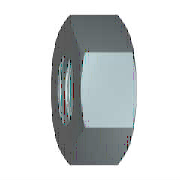
# Autodesk Inventor part: CNS 3129 - M 2
Saved by Autodesk Inventor 2017 (Build 210142000, 142)
## iProperties
IsCustomPart: 0
Created: 2016-02-22
Part Number: CNS 3129 - M 2
Material: Steel, Mild
Description: Hex Nut
Document SubType Name: Modeling
Standard: CNS 3129
Designer: Admin
Standards Organization: CNS
Language: en-US
Size Designation: M 2
Categories: <MemberInstance><Categories><Category DisplayName="Fasteners" InternalName="e4da775c-781d-43d5-af7c-5136215cf5a6" Mnemonic="FSTN"><Category DisplayName="Nuts" InternalName="e37c7a56-0470-4688-8db4-b4d75d611516" Mnemonic="NUT"><CategoryParameter DisplayName="Thread Designation" InternalName="10aefdba-3783-44b8-becc-0feae870ab73" Mnemonic="thrdesign"/><CategoryParameter DisplayName="Thread Series Designation" InternalName="17a0ae10-6923-48a9-85c7-ae9b76790e6f" Mnemonic="thrserdsgn"/><CategoryParameter DisplayName="Thread Type" InternalName="205c6614-02f1-43b1-b704-b331415a8186" Mnemonic="thrtype"/><CategoryParameter DisplayName="Nominal Diameter Designation" InternalName="39406bc0-754a-4a9f-8c64-e1bba9d40b8a" Mnemonic="nomdiadesig"/><CategoryParameter DisplayName="Height" InternalName="5579c84d-d692-41f2-8996-171d03c19b53" Mnemonic="nheig"/><CategoryParameter DisplayName="Thread Class" InternalName="9b95427d-7bb5-461a-8a3e-4650073a592b" Mnemonic="thrclss"/><CategoryParameter DisplayName="Thread Pitch" InternalName="bd2c58b1-df6d-45e3-8bf7-4a0997b15b95" Mnemonic="pitch1"/><CategoryParameter DisplayName="Nominal Diameter" InternalName="d6e3b243-37ab-4432-98ea-592d296d3a46" Mnemonic="nomdia"/><CategoryParameter DisplayName="Threads per Unit" InternalName="e2e4d09d-bc7f-4af6-8086-8693b8d97bcd" Mnemonic="thrperunit1"/><Category DisplayName="Hex" InternalName="73d9c703-2233-4460-907f-38a87f245fbb" Mnemonic="PLNUT"><CategoryParameter DisplayName="Width Across Corners" InternalName="3db1d29f-9506-4e4b-a66f-416ec1d0915f" Mnemonic="wacor"/><CategoryParameter DisplayName="Type" InternalName="4e484966-9917-44a5-bcb5-b45bf8fff7e8" Mnemonic="type"/><CategoryParameter DisplayName="Property Class" InternalName="bcb84129-2a2e-4fb9-8398-d46bb849f471" Mnemonic="propclss"/></Category></Category></Category><Category DisplayName="DataType" InternalName="23b78d0f-2648-40c6-8793-ca6db495c9e8" Mnemonic="DATATYPE"><CategoryParameter DisplayName="DisplayName" InternalName="05415f3d-3907-474b-a020-eb9d644f4cf3" Mnemonic="DISPLAYNAME"/><CategoryParameter DisplayName="Standard" InternalName="0c0a119c-1e12-4c84-803f-101930972f5e" Mnemonic="STANDARD"/><CategoryParameter DisplayName="Description" InternalName="13903e3d-64b1-4950-80da-f627842ea37f" Mnemonic="DESCRIPTION"/><CategoryParameter DisplayName="Designation" InternalName="2675968c-4ce5-49e0-a4f5-552d29089031" Mnemonic="DESIGNATION"/><CategoryParameter DisplayName="Default Row" InternalName="2af9ec52-faaa-4026-b378-f9fa4afca842" Mnemonic="DEFAULTROW"/><CategoryParameter DisplayName="Folder Name" InternalName="3f06958e-8713-4116-9be7-ed6184ecc97b" Mnemonic="FOLDERNAME"/><CategoryParameter DisplayName="Revision Guid" InternalName="45a75005-10b1-4dfc-8d6d-dfe629f0b93c" Mnemonic="REVISIONGUID"/><CategoryParameter DisplayName="FileName" InternalName="8b46a4cc-9585-4fed-90c3-899f57e09a73" Mnemonic="FILENAME"/><CategoryParameter DisplayName="StdsOrg" InternalName="8f5914e1-4693-403f-8ab5-d37768198c9d" Mnemonic="STDSORG"/><CategoryParameter DisplayName="Family Version" InternalName="914462f6-6e19-4b14-ba84-155b9680b1d0" Mnemonic="FAMILYREVISION"/><CategoryParameter DisplayName="Standard Revision" InternalName="91d5a463-65c2-4fde-b823-3b7fea5e8e17" Mnemonic="STANDARDREVISION"/><CategoryParameter DisplayName="Member Revision" InternalName="a65d44b9-392f-4f4f-857b-e4b3d54996fe" Mnemonic="MEMBERREVISION"/><CategoryParameter DisplayName="ClipFormat" InternalName="bc51e27b-3422-4e78-93ef-cec197ddf230" Mnemonic="CLIPFORMAT"/><CategoryParameter DisplayName="Manufacturer" InternalName="cd6c7a72-a28a-4e50-99a9-2c7f4e13e5ad" Mnemonic="MANUFACTURER"/><CategoryParameter DisplayName="InternalName" InternalName="cf1d0246-76d9-4b4a-8305-fa0409afb5c1" Mnemonic="INTERNALNAME"/><CategoryParameter DisplayName="IsMetric" InternalName="e2385c5b-1ea4-4823-96a8-8de651266ec3" Mnemonic="ISMETRIC"/><Category DisplayName="Part" InternalName="c0e0b642-3bcb-4cc8-9e80-f96d35c4afa4" Mnemonic="PART"><CategoryParameter DisplayName="Part Number" InternalName="016b6077-bfbe-49bd-92c9-d8d59c39c941" Mnemonic="PARTNUMBER"/><CategoryParameter DisplayName="Stock Number" InternalName="4dba7c1c-e26c-444e-836c-b08b433409a8" Mnemonic="STOCKNUMBER"/><CategoryParameter DisplayName="Material Key" InternalName="5c9a8adb-dd2b-4535-b97f-0a94a95fe41f" Mnemonic="MATERIALKEY"/><CategoryParameter DisplayName="Material" InternalName="818a152a-d3c3-49ca-80ee-df7d91421b8e" Mnemonic="MATERIAL"/></Category></Category><Category DisplayName="LegacyMap" InternalName="cd87c42b-3e48-431e-b5c0-1cbeb14dfe77" Mnemonic="LEGACYMAP"><CategoryParameter DisplayName="unique DA member ID" InternalName="0918ad47-427f-4fed-ae26-24c81c58f590" Mnemonic="DACOOKIE"/><CategoryParameter DisplayName="Merge11 ID" InternalName="0ee8fb18-e2ed-4f39-96f6-1f4b5f50aa71" Mnemonic="MERGE11"/><CategoryParameter DisplayName="unique CC member ID" InternalName="5193edd4-b2b0-4ab4-9d54-de900eee34e0" Mnemonic="CCCOOKIE"/><CategoryParameter DisplayName="Split ID" InternalName="72b5c83c-be7f-45c4-ae51-9160ea6deb26" Mnemonic="SPLIT"/><CategoryParameter DisplayName="MemberID" InternalName="8e5e0294-fc51-4c8f-b3d7-003dc5ed94f6" Mnemonic="MEMBERID"/><CategoryParameter DisplayName="CatalogName" InternalName="d99d1e27-aa94-4de2-af4c-c348882a6f4f" Mnemonic="CATALOGNAME"/><CategoryParameter DisplayName="FamilyNumber" InternalName="e705e1f4-09cb-413e-91f9-551b4188271e" Mnemonic="FAMILYNUMBER"/></Category></Categories><FamilyTemplate Id="no0010"><FamilyTemplateParameters><FamilyTemplateParameter ObjectType="kUserParameterObject" ValueType="xs:double" Id="1" ObjectReferenceKey="GUL"/><FamilyTemplateParameter ObjectType="kUserParameterObject" ValueType="xs:double" Id="2" ObjectReferenceKey="KOH"/><FamilyTemplateParameter ObjectType="kUserParameterObject" ValueType="xs:double" Id="3" ObjectReferenceKey="TPU"/><FamilyTemplateParameter ObjectType="kUserParameterObject" ValueType="xs:double" Id="4" ObjectReferenceKey="GD1"/><FamilyTemplateParameter ObjectType="kUserParameterObject" ValueType="xs:double" Id="5" ObjectReferenceKey="SW01"/><FamilyTemplateParameter ObjectType="kUserParameterObject" ValueType="xs:double" Id="6" ObjectReferenceKey="THREADDIA"/><FamilyTemplateParameter ObjectType="kUserParameterObject" ValueType="xs:double" Id="7" ObjectReferenceKey="SW"/><FamilyTemplateParameter ObjectType="kUserParameterObject" ValueType="xs:double" Id="8" ObjectReferenceKey="ANG2"/><FamilyTemplateParameter ObjectType="kUserParameterObject" ValueType="xs:double" Id="9" ObjectReferenceKey="ANG1"/><FamilyTemplateParameter ObjectType="kUserParameterObject" ValueType="xs:double" Id="10" ObjectReferenceKey="TOA"/><FamilyTemplateParameter ObjectType="kUserParameterObject" ValueType="xs:double" Id="11" ObjectReferenceKey="PTC"/><FamilyTemplateParameter ObjectType="kUserParameterObject" ValueType="xs:double" Id="12" ObjectReferenceKey="NND"/><FamilyTemplateParameter ObjectType="kUserParameterObject" ValueType="xs:double" Id="13" ObjectReferenceKey="E0"/><FamilyTemplateParameter ObjectType="kUserParameterObject" ValueType="xs:double" Id="14" ObjectReferenceKey="SW0"/><FamilyTemplateParameter ObjectType="kUserParameterObject" ValueType="xs:double" Id="15" ObjectReferenceKey="GAL"/><FamilyTemplateParameter ObjectType="kPropertyObject" ValueType="xs:string" Id="100" ObjectReferenceKey="{32853F0F-3444-11d1-9E93-0060B03C1CA6}" SubObjectId="52"/><FamilyTemplateParameter ObjectType="kPropertyObject" ValueType="xs:string" Id="105" ObjectReferenceKey="{32853F0F-3444-11d1-9E93-0060B03C1CA6}" SubObjectId="5"/><FamilyTemplateParameter ObjectType="kPartComponentDefinitionObject" ValueType="xs:string" Id="110" SubObjectId="Material"/><FamilyTemplateParameter ObjectType="kThreadFeatureObject" ValueType="xs:structure" Id="300" ObjectReferenceKey="1002000010000000ba090000000000008000000000000000" SubObjectId="ThreadInfo"><FamilyTemplateParameter ObjectType="" ValueType="xs:string" Id="301" SubObjectId="ThreadDesignation"/><FamilyTemplateParameter ObjectType="" ValueType="xs:string" Id="302" SubObjectId="ThreadClass"/><FamilyTemplateParameter ObjectType="" ValueType="xs:string" Id="303" SubObjectId="ThreadType"/></FamilyTemplateParameter></FamilyTemplateParameters></FamilyTemplate><CategoryParameterMap><ParamToTemplateMap><ParamToTemplate CategoryParameter="//CategoryParameter[@InternalName='05415f3d-3907-474b-a020-eb9d644f4cf3']" ConstantValue="CNS 3129"/><ParamToTemplate CategoryParameter="//CategoryParameter[@InternalName='cf1d0246-76d9-4b4a-8305-fa0409afb5c1']" ConstantValue="5d0b1584-d28e-4f5c-b995-5fb680a39008"/><ParamToTemplate CategoryParameter="//CategoryParameter[@InternalName='3f06958e-8713-4116-9be7-ed6184ecc97b']" ConstantValue="CNS 3129"/><ParamToTemplate CategoryParameter="//CategoryParameter[@InternalName='914462f6-6e19-4b14-ba84-155b9680b1d0']" ConstantValue="10"/><ParamToTemplate CategoryParameter="//CategoryParameter[@InternalName='bc51e27b-3422-4e78-93ef-cec197ddf230']" ConstantValue="CF_INVENTOR.STDPARTS"/><ParamToTemplate CategoryParameter="//CategoryParameter[@InternalName='e2385c5b-1ea4-4823-96a8-8de651266ec3']" ConstantValue="true"/><ParamToTemplate CategoryParameter="//CategoryParameter[@InternalName='13903e3d-64b1-4950-80da-f627842ea37f']" ConstantValue="Hex Nut"/><ParamToTemplate CategoryParameter="//CategoryParameter[@InternalName='8f5914e1-4693-403f-8ab5-d37768198c9d']" ConstantValue="CNS"/><ParamToTemplate CategoryParameter="//CategoryParameter[@InternalName='0c0a119c-1e12-4c84-803f-101930972f5e']" ConstantValue="CNS 3129"/><ParamToTemplate CategoryParameter="//CategoryParameter[@InternalName='cd6c7a72-a28a-4e50-99a9-2c7f4e13e5ad']" TemplateParameter="104"/><ParamToTemplate CategoryParameter="//CategoryParameter[@InternalName='91d5a463-65c2-4fde-b823-3b7fea5e8e17']" TemplateParameter="103"/><ParamToTemplate CategoryParameter="//CategoryParameter[@InternalName='45a75005-10b1-4dfc-8d6d-dfe629f0b93c']" ConstantValue="ca1287fc-ef04-4131-a459-e0ad3082d8c4"/><ParamToTemplate CategoryParameter="//CategoryParameter[@InternalName='2af9ec52-faaa-4026-b378-f9fa4afca842']" ConstantValue="10"/><ParamToTemplate CategoryParameter="//CategoryParameter[@InternalName='d99d1e27-aa94-4de2-af4c-c348882a6f4f']" ConstantValue="CNS"/><ParamToTemplate CategoryParameter="//CategoryParameter[@InternalName='8b46a4cc-9585-4fed-90c3-899f57e09a73']" ConstantValue="CNS 3129 - M 2 x 0.4"/><ParamToTemplate CategoryParameter="//CategoryParameter[@InternalName='a65d44b9-392f-4f4f-857b-e4b3d54996fe']" ConstantValue="a0c9818c-55a9-4959-93a9-f48d9538dd43"/><ParamToTemplate CategoryParameter="//CategoryParameter[@InternalName='9b95427d-7bb5-461a-8a3e-4650073a592b']" ConstantValue="6H"/><ParamToTemplate CategoryParameter="//CategoryParameter[@InternalName='17a0ae10-6923-48a9-85c7-ae9b76790e6f']" ConstantValue="Regular Thread"/><ParamToTemplate CategoryParameter="//CategoryParameter[@InternalName='39406bc0-754a-4a9f-8c64-e1bba9d40b8a']" ConstantValue="M2"/><ParamToTemplate CategoryParameter="//CategoryParameter[@InternalName='205c6614-02f1-43b1-b704-b331415a8186']" ConstantValue="ISO Metric Profile"/><ParamToTemplate CategoryParameter="//CategoryParameter[@InternalName='e705e1f4-09cb-413e-91f9-551b4188271e']" ConstantValue="53"/><ParamToTemplate CategoryParameter="//CategoryParameter[@InternalName='8e5e0294-fc51-4c8f-b3d7-003dc5ed94f6']" ConstantValue="30"/><ParamToTemplate CategoryParameter="//CategoryParameter[@InternalName='2675968c-4ce5-49e0-a4f5-552d29089031']" TemplateParameter="100"/><ParamToTemplate CategoryParameter="//CategoryParameter[@InternalName='3db1d29f-9506-4e4b-a66f-416ec1d0915f']" TemplateParameter="13"/><ParamToTemplate CategoryParameter="//CategoryParameter[@InternalName='5579c84d-d692-41f2-8996-171d03c19b53']" TemplateParameter="2"/><ParamToTemplate CategoryParameter="//CategoryParameter[@InternalName='818a152a-d3c3-49ca-80ee-df7d91421b8e']" TemplateParameter="110"/><ParamToTemplate CategoryParameter="//CategoryParameter[@InternalName='d6e3b243-37ab-4432-98ea-592d296d3a46']" TemplateParameter="12"/><ParamToTemplate CategoryParameter="//CategoryParameter[@InternalName='016b6077-bfbe-49bd-92c9-d8d59c39c941']" TemplateParameter="105"/><ParamToTemplate CategoryParameter="//CategoryParameter[@InternalName='bd2c58b1-df6d-45e3-8bf7-4a0997b15b95']" TemplateParameter="11"/><ParamToTemplate CategoryParameter="//CategoryParameter[@InternalName='10aefdba-3783-44b8-becc-0feae870ab73']" TemplateParameter="301"/><ParamToTemplate CategoryParameter="//CategoryParameter[@InternalName='e2e4d09d-bc7f-4af6-8086-8693b8d97bcd']" TemplateParameter="3"/></ParamToTemplateMap></CategoryParameterMap></MemberInstance>
Density: 7.85 g/cm^3
Appearance: Semi-Polished
Mass: 0.110128 g
Surface Area: 0.442366 cm^2
Volume: 0.014029 cm^3
Author: Admin
Autodesk Inventor part; units mm, degrees
ref_plane "YZ Plane" through (0, 0, 0) normal (1, 0, 0) x (0, 1, 0)
ref_plane "XZ Plane" through (0, 0, 0) normal (0, 1, 0) x (-1, 0, 0)
sketch "Sketch1" plane through (0, 0, 0) normal (1, 0, 0) x (0, 1, 0)
  line L0 (-2.3094, 0) -> (-1.1547, 2)
  line L1 (-1.1547, 2) -> (1.1547, 2)
  line L2 (1.1547, 2) -> (2.3094, 0)
  line L3 (2.3094, 0) -> (1.1547, -2)
  line L4 (1.1547, -2) -> (-1.1547, -2)
  line L5 (-1.1547, -2) -> (-2.3094, 0)
  point P0 (0, 0)
  point P1 (0, 0)
  dimension "d0" = 4.6188
  constraints: 12 end point, 1 coincident, 1 horizontal, 11 other
  measures "d0" distance of L2.end L0.start
extrude "Body" add sketch "Sketch1" along normal blind 1.2
sketch "Sketch2" plane through (0, 0, 0) normal (0, 0, 1) x (1, 0, 0)
  line L0 (0, 1.1547) -> (0, 2.3094) projected
  line L1 (0, 2.3094) -> (1.2, 2.3094) projected
  line L2 (1.2, 1.1547) -> (1.2, 2.3094) projected
  line L3 (-0.24, 0) -> (1.44, 0) projected
  line L4 (0.1786, 2.3094) -> (0, 2)
  line L5 (1.0214, 2.3094) -> (1.2, 2)
  dimension "d3" = 30
  dimension "d4" = 30
  dimension "d5" = 4
  dimension "d6" = 4
  constraints: 4 end point, 4 point on line
  measures "d3" angle of L0 L4
  measures "d4" angle of L2 L5
  measures "d5" diameter of L4.end L3
  measures "d6" diameter of L5.end L3
revolve "Chamfer1" cut sketch "Sketch2" angle 360 about axis through (-10, 0, 0) along (1, 0, 0)
sketch "Sketch3" plane through (1.2, 0, 0) normal (1, 0, 0) x (0, 0, -1)
  arc A0 (-1, -1.7321) -> (1, -1.7321) centre (0, 0) ccw projected
  constraints: 1 coincident
hole "Thread" at (1.2, 0, 0) direction (-1, 0, 0) diameter 1.567 end through all thread size "M2x0.4" class "6H" standard "ISO Metric profile"
chamfer "Chamfer2" distance 0.2165 angle 30 1 edges at (1.2, 0, 0.7835) measured on face at (1.2, 1.5853, -0.0315)
chamfer "Chamfer3" distance 0.2165 angle 30 1 edges at (0, 0, 0.7835) measured on face at (0, 1.5853, -0.0315)
ref_plane "Work Plane1" through (-5.0268, 0, 0) normal (0, -0.866, -0.5) x (1, 0, 0)
equation "\"d0\" = 1.1547 * SW"
equation "\"d1\" = KOH"
equation "\"d3\" = ANG1"
equation "\"d4\" = ANG2"
equation "\"d5\" = SW0"
equation "\"d6\" = SW01"
equation "\"d8\" = -0.5 * GD1 + 0.5 * NND"
equation "\"d40\" = -0.5 * GD1 + 0.5 * NND"
equation "\"d10\" = -0.5 * GD1 + 0.5 * NND"
equation "\"d41\" = -0.5 * GD1 + 0.5 * NND"
equation "\"ANG1\" = 30deg"
equation "\"ANG2\" = 30deg"
equation "\"NND\" = 2"
equation "\"KOH\" = 1.2"
equation "\"SW\" = 4"
equation "\"SW0\" = SW"
equation "\"SW01\" = SW"
equation "\"GUL\" = 0.541266 * PTC"
equation "\"THREADDIA\" = 2"
equation "\"TOA\" = 30deg"
equation "\"PTC\" = 0.4"
equation "\"E0\" = 1.155 * SW"
equation "\"GAL\" = 0.541266 * PTC"
equation "\"GD1\" = 1.566987"
body "Solid1"
